Autodesk Fusion 360 part; units mm, degrees
(part 8 of 9)
equation "d1459 = ( BaseX ) + ( Wall + DeckClearance + RimBorder )"
equation "d1460 = ( BaseY + Depth + ModuleGap ) + ( ( LeftReach ) - ( ( ( ( ( LeftReach ) - ( 14 * SlotPitch + SlotWidth ) ) / 2 ) + ( 5 * SlotPitch ) ) + ( SlotWidth ) ) )"
equation "d1461 = ( LeftSideDepth ) - 2 * ( Wall + DeckClearance + RimBorder )"
equation "d1462 = SlotWidth"
equation "d1463 = DeckThick"
equation "d1465 = ( FootHeight ) + PanHeight - DeckThick"
equation "d1467 = ( BaseX ) + ( Wall + DeckClearance + RimBorder )"
equation "d1468 = ( BaseY + Depth + ModuleGap ) + ( ( LeftReach ) - ( ( ( ( ( LeftReach ) - ( 14 * SlotPitch + SlotWidth ) ) / 2 ) + ( 6 * SlotPitch ) ) + ( SlotWidth ) ) )"
equation "d1469 = ( LeftSideDepth ) - 2 * ( Wall + DeckClearance + RimBorder )"
equation "d1470 = SlotWidth"
equation "d1471 = DeckThick"
equation "d1473 = ( FootHeight ) + PanHeight - DeckThick"
equation "d1475 = ( BaseX ) + ( Wall + DeckClearance + RimBorder )"
equation "d1476 = ( BaseY + Depth + ModuleGap ) + ( ( LeftReach ) - ( ( ( ( ( LeftReach ) - ( 14 * SlotPitch + SlotWidth ) ) / 2 ) + ( 7 * SlotPitch ) ) + ( SlotWidth ) ) )"
equation "d1477 = ( LeftSideDepth ) - 2 * ( Wall + DeckClearance + RimBorder )"
equation "d1478 = SlotWidth"
equation "d1479 = DeckThick"
equation "d1481 = ( FootHeight ) + PanHeight - DeckThick"
equation "d1483 = ( BaseX ) + ( Wall + DeckClearance + RimBorder )"
equation "d1484 = ( BaseY + Depth + ModuleGap ) + ( ( LeftReach ) - ( ( ( ( ( LeftReach ) - ( 14 * SlotPitch + SlotWidth ) ) / 2 ) + ( 8 * SlotPitch ) ) + ( SlotWidth ) ) )"
equation "d1485 = ( LeftSideDepth ) - 2 * ( Wall + DeckClearance + RimBorder )"
equation "d1486 = SlotWidth"
equation "d1487 = DeckThick"
equation "d1489 = ( FootHeight ) + PanHeight - DeckThick"
equation "d1491 = ( BaseX ) + ( Wall + DeckClearance + RimBorder )"
equation "d1492 = ( BaseY + Depth + ModuleGap ) + ( ( LeftReach ) - ( ( ( ( ( LeftReach ) - ( 14 * SlotPitch + SlotWidth ) ) / 2 ) + ( 9 * SlotPitch ) ) + ( SlotWidth ) ) )"
equation "d1493 = ( LeftSideDepth ) - 2 * ( Wall + DeckClearance + RimBorder )"
equation "d1494 = SlotWidth"
equation "d1495 = DeckThick"
equation "d1497 = ( FootHeight ) + PanHeight - DeckThick"
equation "d1499 = ( BaseX ) + ( Wall + DeckClearance + RimBorder )"
equation "d1500 = ( BaseY + Depth + ModuleGap ) + ( ( LeftReach ) - ( ( ( ( ( LeftReach ) - ( 14 * SlotPitch + SlotWidth ) ) / 2 ) + ( 10 * SlotPitch ) ) + ( SlotWidth ) ) )"
equation "d1501 = ( LeftSideDepth ) - 2 * ( Wall + DeckClearance + RimBorder )"
equation "d1502 = SlotWidth"
equation "d1503 = DeckThick"
equation "d1505 = ( FootHeight ) + PanHeight - DeckThick"
equation "d1507 = ( BaseX ) + ( Wall + DeckClearance + RimBorder )"
equation "d1508 = ( BaseY + Depth + ModuleGap ) + ( ( LeftReach ) - ( ( ( ( ( LeftReach ) - ( 14 * SlotPitch + SlotWidth ) ) / 2 ) + ( 11 * SlotPitch ) ) + ( SlotWidth ) ) )"
equation "d1509 = ( LeftSideDepth ) - 2 * ( Wall + DeckClearance + RimBorder )"
equation "d1510 = SlotWidth"
equation "d1511 = DeckThick"
equation "d1513 = ( FootHeight ) + PanHeight - DeckThick"
equation "d1515 = ( BaseX ) + ( Wall + DeckClearance + RimBorder )"
equation "d1516 = ( BaseY + Depth + ModuleGap ) + ( ( LeftReach ) - ( ( ( ( ( LeftReach ) - ( 14 * SlotPitch + SlotWidth ) ) / 2 ) + ( 12 * SlotPitch ) ) + ( SlotWidth ) ) )"
equation "d1517 = ( LeftSideDepth ) - 2 * ( Wall + DeckClearance + RimBorder )"
equation "d1518 = SlotWidth"
equation "d1519 = DeckThick"
equation "d1521 = ( FootHeight ) + PanHeight - DeckThick"
equation "d1523 = ( BaseX ) + ( Wall + DeckClearance + RimBorder )"
equation "d1524 = ( BaseY + Depth + ModuleGap ) + ( ( LeftReach ) - ( ( ( ( ( LeftReach ) - ( 14 * SlotPitch + SlotWidth ) ) / 2 ) + ( 13 * SlotPitch ) ) + ( SlotWidth ) ) )"
equation "d1525 = ( LeftSideDepth ) - 2 * ( Wall + DeckClearance + RimBorder )"
equation "d1526 = SlotWidth"
equation "d1527 = DeckThick"
equation "d1529 = ( FootHeight ) + PanHeight - DeckThick"
equation "d1531 = ( BaseX ) + ( Wall + DeckClearance + RimBorder )"
equation "d1532 = ( BaseY + Depth + ModuleGap ) + ( ( LeftReach ) - ( ( ( ( ( LeftReach ) - ( 14 * SlotPitch + SlotWidth ) ) / 2 ) + ( 14 * SlotPitch ) ) + ( SlotWidth ) ) )"
equation "d1533 = ( LeftSideDepth ) - 2 * ( Wall + DeckClearance + RimBorder )"
equation "d1534 = SlotWidth"
equation "d1535 = DeckThick"
equation "d1537 = ( FootHeight ) + PanHeight - DeckThick"
equation "d1539 = ( BaseX ) + ( ( LeftSideDepth ) - Wall - DeckClearance - 4 mm )"
equation "d1540 = ( BaseY + Depth + ModuleGap ) + ( ( LeftReach ) - ( ( ( LeftReach ) / 2 - 8 mm ) + ( 16 mm ) ) )"
equation "d1543 = DeckThick"
equation "d1547 = ( BaseX ) + ( ( 11 mm ) - FootSize / 2 )"
equation "d1548 = ( BaseY + Depth + ModuleGap ) + ( ( LeftReach ) - ( ( ( 11 mm ) - FootSize / 2 ) + ( FootSize ) ) )"
equation "d1549 = FootSize"
equation "d1550 = FootSize"
equation "d1551 = FootHeight"
equation "d1553 = FootHeight"
equation "d1555 = ( BaseX ) + ( ( 11 mm ) - PegSize / 2 )"
equation "d1556 = ( BaseY + Depth + ModuleGap ) + ( ( LeftReach ) - ( ( ( 11 mm ) - PegSize / 2 ) + ( PegSize ) ) )"
equation "d1557 = PegSize"
equation "d1558 = PegSize"
equation "d1559 = PegHeight"
equation "d1563 = ( BaseX ) + ( ( ( LeftSideDepth ) - FrontFootInset ) - FootSize / 2 )"
equation "d1564 = ( BaseY + Depth + ModuleGap ) + ( ( LeftReach ) - ( ( ( 11 mm ) - FootSize / 2 ) + ( FootSize ) ) )"
equation "d1565 = FootSize"
equation "d1566 = FootSize"
equation "d1567 = FootHeight"
equation "d1569 = FootHeight"
equation "d1571 = ( BaseX ) + ( ( ( LeftSideDepth ) - FrontFootInset ) - PegSize / 2 )"
equation "d1572 = ( BaseY + Depth + ModuleGap ) + ( ( LeftReach ) - ( ( ( 11 mm ) - PegSize / 2 ) + ( PegSize ) ) )"
equation "d1573 = PegSize"
equation "d1574 = PegSize"
equation "d1575 = PegHeight"
equation "d1579 = ( BaseX ) + ( ( 11 mm ) - FootSize / 2 )"
equation "d1580 = ( BaseY + Depth + ModuleGap ) + ( ( LeftReach ) - ( ( ( ( LeftReach ) - 11 mm ) - FootSize / 2 ) + ( FootSize ) ) )"
equation "d1581 = FootSize"
equation "d1582 = FootSize"
equation "d1583 = FootHeight"
equation "d1585 = FootHeight"
equation "d1587 = ( BaseX ) + ( ( 11 mm ) - PegSize / 2 )"
equation "d1588 = ( BaseY + Depth + ModuleGap ) + ( ( LeftReach ) - ( ( ( ( LeftReach ) - 11 mm ) - PegSize / 2 ) + ( PegSize ) ) )"
equation "d1589 = PegSize"
equation "d1590 = PegSize"
equation "d1591 = PegHeight"
equation "d1595 = ( BaseX ) + ( ( ( LeftSideDepth ) - FrontFootInset ) - FootSize / 2 )"
equation "d1596 = ( BaseY + Depth + ModuleGap ) + ( ( LeftReach ) - ( ( ( ( LeftReach ) - 11 mm ) - FootSize / 2 ) + ( FootSize ) ) )"
equation "d1597 = FootSize"
equation "d1598 = FootSize"
equation "d1599 = FootHeight"
equation "d1601 = FootHeight"
equation "d1603 = ( BaseX ) + ( ( ( LeftSideDepth ) - FrontFootInset ) - PegSize / 2 )"
equation "d1604 = ( BaseY + Depth + ModuleGap ) + ( ( LeftReach ) - ( ( ( ( LeftReach ) - 11 mm ) - PegSize / 2 ) + ( PegSize ) ) )"
equation "d1605 = PegSize"
equation "d1606 = PegSize"
equation "d1607 = PegHeight"
equation "d1609 = FootHeight"
equation "d1611 = ( BaseX + LeftRun + FaucetGap + RightRun - RightSideDepth ) + ( ( RightSideDepth ) - ( ( 0 mm ) + ( RightSideDepth ) ) )"
equation "d1612 = ( BaseY + Depth + ModuleGap ) + ( 0 mm )"
equation "d1613 = RightSideDepth"
equation "d1614 = RightReach"
equation "d1615 = PanHeight"
equation "d1619 = ( BaseY + Depth + ModuleGap ) + ( Wall )"
equation "d1621 = ( ( BaseX + LeftRun + FaucetGap + RightRun - RightSideDepth ) + ( ( RightSideDepth ) - ( Wall ) ) )"
equation "d1622 = -( -( ( FootHeight ) + FloorMin + DrainExtension * tan(DrainSlope) + ( ( RightSideDepth ) - ( Wall ) ) * tan(DrainSlope) ) )"
equation "d1623 = ( ( BaseX + LeftRun + FaucetGap + RightRun - RightSideDepth ) + ( ( RightSideDepth ) - ( ( RightSideDepth ) - Wall ) ) )"
equation "d1624 = -( -( ( FootHeight ) + FloorMin + DrainExtension * tan(DrainSlope) + ( ( RightSideDepth ) - ( ( RightSideDepth ) - Wall ) ) * tan(DrainSlope) ) )"
equation "d1625 = -( -( ( FootHeight ) + PanHeight + 1 mm ) )"
equation "d1626 = ( RightReach ) - 2 * Wall"
equation "d1628 = ( BaseY + Depth + ModuleGap ) + ( ( RightReach / 2 ) - DrainWidth / 2 - Wall )"
equation "d1630 = ( ( BaseX + LeftRun + FaucetGap + RightRun - RightSideDepth ) + ( ( RightSideDepth ) - ( ( RightSideDepth ) - Wall ) ) )"
equation "d1631 = -( -( FootHeight ) )"
equation "d1632 = ( ( BaseX + LeftRun + FaucetGap + RightRun - RightSideDepth ) + ( ( RightSideDepth ) - ( ( RightSideDepth ) + DrainExtension ) ) )"
equation "d1633 = -( -( ( FootHeight ) + FloorMin + DrainExtension * tan(DrainSlope) + ( ( RightSideDepth ) - ( ( RightSideDepth ) + DrainExtension ) ) * tan(DrainSlope) ) )"
equation "d1634 = -( -( ( FootHeight ) + FloorMin + DrainExtension * tan(DrainSlope) + ( ( RightSideDepth ) - ( ( RightSideDepth ) - Wall ) ) * tan(DrainSlope) ) )"
equation "d1635 = DrainWidth + 2 * Wall"
equation "d1637 = ( BaseY + Depth + ModuleGap ) + ( ( RightReach / 2 ) - DrainWidth / 2 - Wall )"
equation "d1639 = ( ( BaseX + LeftRun + FaucetGap + RightRun - RightSideDepth ) + ( ( RightSideDepth ) - ( ( RightSideDepth ) - Wall ) ) )"
equation "d1640 = -( -( FootHeight ) )"
equation "d1641 = ( ( BaseX + LeftRun + FaucetGap + RightRun - RightSideDepth ) + ( ( RightSideDepth ) - ( ( RightSideDepth ) + DrainExtension ) ) )"
equation "d1642 = -( -( ( ( FootHeight ) + FloorMin + DrainExtension * tan(DrainSlope) + ( ( RightSideDepth ) - ( ( RightSideDepth ) + DrainExtension ) ) * tan(DrainSlope) ) + ( 6 mm ) ) )"
equation "d1643 = -( -( ( ( FootHeight ) + FloorMin + DrainExtension * tan(DrainSlope) + ( ( RightSideDepth ) - ( ( RightSideDepth ) - Wall ) ) * tan(DrainSlope) ) + ( 6 mm ) ) )"
equation "d1644 = Wall"
equation "d1646 = ( BaseY + Depth + ModuleGap ) + ( ( RightReach / 2 ) + DrainWidth / 2 )"
equation "d1648 = ( ( BaseX + LeftRun + FaucetGap + RightRun - RightSideDepth ) + ( ( RightSideDepth ) - ( ( RightSideDepth ) - Wall ) ) )"
equation "d1649 = -( -( FootHeight ) )"
equation "d1650 = ( ( BaseX + LeftRun + FaucetGap + RightRun - RightSideDepth ) + ( ( RightSideDepth ) - ( ( RightSideDepth ) + DrainExtension ) ) )"
equation "d1651 = -( -( ( ( FootHeight ) + FloorMin + DrainExtension * tan(DrainSlope) + ( ( RightSideDepth ) - ( ( RightSideDepth ) + DrainExtension ) ) * tan(DrainSlope) ) + ( 6 mm ) ) )"
equation "d1652 = -( -( ( ( FootHeight ) + FloorMin + DrainExtension * tan(DrainSlope) + ( ( RightSideDepth ) - ( ( RightSideDepth ) - Wall ) ) * tan(DrainSlope) ) + ( 6 mm ) ) )"
equation "d1653 = Wall"
equation "d1655 = ( BaseY + Depth + ModuleGap ) + ( ( RightReach / 2 ) - DrainWidth / 2 )"
equation "d1657 = ( ( BaseX + LeftRun + FaucetGap + RightRun - RightSideDepth ) + ( ( RightSideDepth ) - ( ( RightSideDepth ) - Wall ) ) )"
equation "d1658 = -( -( ( FootHeight ) + FloorMin + DrainExtension * tan(DrainSlope) + ( ( RightSideDepth ) - ( ( RightSideDepth ) - Wall ) ) * tan(DrainSlope) ) )"
equation "d1659 = ( ( BaseX + LeftRun + FaucetGap + RightRun - RightSideDepth ) + ( ( RightSideDepth ) - ( ( RightSideDepth ) + DrainExtension ) ) )"
equation "d1660 = -( -( ( FootHeight ) + FloorMin + DrainExtension * tan(DrainSlope) + ( ( RightSideDepth ) - ( ( RightSideDepth ) + DrainExtension ) ) * tan(DrainSlope) ) )"
equation "d1661 = -( -( ( FootHeight ) + PanHeight + 1 mm ) )"
equation "d1662 = DrainWidth"
equation "d1664 = FootHeight"
equation "d1666 = ( BaseX + LeftRun + FaucetGap + RightRun - RightSideDepth ) + ( ( RightSideDepth ) - ( ( Wall ) + ( 12 mm ) ) )"
equation "d1667 = ( BaseY + Depth + ModuleGap ) + ( Wall )"
equation "d1670 = PanHeight - DeckThick"
equation "d1672 = FootHeight"
equation "d1674 = ( BaseX + LeftRun + FaucetGap + RightRun - RightSideDepth ) + ( ( RightSideDepth ) - ( ( ( RightSideDepth ) - Wall - 12 mm ) + ( 12 mm ) ) )"
equation "d1675 = ( BaseY + Depth + ModuleGap ) + ( Wall )"
equation "d1678 = PanHeight - DeckThick"
equation "d1680 = FootHeight"
equation "d1682 = ( BaseX + LeftRun + FaucetGap + RightRun - RightSideDepth ) + ( ( RightSideDepth ) - ( ( Wall ) + ( 12 mm ) ) )"
equation "d1683 = ( BaseY + Depth + ModuleGap ) + ( ( RightReach ) - Wall - 12 mm )"
equation "d1686 = PanHeight - DeckThick"
equation "d1688 = FootHeight"
equation "d1690 = ( BaseX + LeftRun + FaucetGap + RightRun - RightSideDepth ) + ( ( RightSideDepth ) - ( ( ( RightSideDepth ) - Wall - 12 mm ) + ( 12 mm ) ) )"
equation "d1691 = ( BaseY + Depth + ModuleGap ) + ( ( RightReach ) - Wall - 12 mm )"
equation "d1694 = PanHeight - DeckThick"
equation "d1696 = ( BaseY + Depth + ModuleGap ) + ( ( RightReach / 2 ) - DrainWidth / 2 - Wall )"
equation "d1698 = ( ( BaseX + LeftRun + FaucetGap + RightRun - RightSideDepth ) + ( ( RightSideDepth ) - ( ( RightSideDepth ) + DrainExtension - 2 mm ) ) )"
equation "d1699 = -( -( ( FootHeight ) - ( 0.2 mm ) ) )"
equation "d1700 = ( ( BaseX + LeftRun + FaucetGap + RightRun - RightSideDepth ) + ( ( RightSideDepth ) - ( ( ( RightSideDepth ) + DrainExtension - 2 mm ) + ( 1 mm ) ) ) )"
equation "d1701 = -( -( ( FootHeight ) + ( 0.6 mm ) ) )"
equation "d1702 = DrainWidth + 2 * Wall"
equation "d1704 = FootHeight"
equation "d1706 = ( BaseX + LeftRun + FaucetGap + RightRun - RightSideDepth ) + ( ( RightSideDepth ) - ( ( ( 11 mm ) - PegSize / 2 - FitClearance ) + ( PegSize + 2 * FitClearance ) ) )"
equation "d1707 = ( BaseY + Depth + ModuleGap ) + ( ( 11 mm ) - PegSize / 2 - FitClearance )"
equation "d1708 = PegSize + 2 * FitClearance"
equation "d1709 = PegSize + 2 * FitClearance"
equation "d1710 = PegHeight + 0.3 mm"
equation "d1712 = FootHeight"
equation "d1714 = ( BaseX + LeftRun + FaucetGap + RightRun - RightSideDepth ) + ( ( RightSideDepth ) - ( ( ( ( RightSideDepth ) - FrontFootInset ) - PegSize / 2 - FitClearance ) + ( PegSize + 2 * FitClearance ) ) )"
equation "d1715 = ( BaseY + Depth + ModuleGap ) + ( ( 11 mm ) - PegSize / 2 - FitClearance )"
equation "d1716 = PegSize + 2 * FitClearance"
equation "d1717 = PegSize + 2 * FitClearance"
equation "d1718 = PegHeight + 0.3 mm"
equation "d1720 = FootHeight"
equation "d1722 = ( BaseX + LeftRun + FaucetGap + RightRun - RightSideDepth ) + ( ( RightSideDepth ) - ( ( ( 11 mm ) - PegSize / 2 - FitClearance ) + ( PegSize + 2 * FitClearance ) ) )"
equation "d1723 = ( BaseY + Depth + ModuleGap ) + ( ( ( RightReach ) - 11 mm ) - PegSize / 2 - FitClearance )"
equation "d1724 = PegSize + 2 * FitClearance"
equation "d1725 = PegSize + 2 * FitClearance"
equation "d1726 = PegHeight + 0.3 mm"
equation "d1728 = FootHeight"
equation "d1730 = ( BaseX + LeftRun + FaucetGap + RightRun - RightSideDepth ) + ( ( RightSideDepth ) - ( ( ( ( RightSideDepth ) - FrontFootInset ) - PegSize / 2 - FitClearance ) + ( PegSize + 2 * FitClearance ) ) )"
equation "d1731 = ( BaseY + Depth + ModuleGap ) + ( ( ( RightReach ) - 11 mm ) - PegSize / 2 - FitClearance )"
equation "d1732 = PegSize + 2 * FitClearance"
equation "d1733 = PegSize + 2 * FitClearance"
equation "d1734 = PegHeight + 0.3 mm"
equation "d1736 = ( FootHeight ) + PanHeight - DeckThick"
equation "d1738 = ( BaseX + LeftRun + FaucetGap + RightRun - RightSideDepth ) + ( ( RightSideDepth ) - ( ( Wall + DeckClearance ) + ( ( RightSideDepth ) - 2 * ( Wall + DeckClearance ) ) ) )"
equation "d1739 = ( BaseY + Depth + ModuleGap ) + ( Wall + DeckClearance )"
equation "d1740 = ( RightSideDepth ) - 2 * ( Wall + DeckClearance )"
equation "d1741 = ( RightReach ) - 2 * ( Wall + DeckClearance )"
equation "d1742 = DeckThick"
equation "d1744 = ( FootHeight ) + PanHeight - DeckThick"
equation "d1746 = ( BaseX + LeftRun + FaucetGap + RightRun - RightSideDepth ) + ( ( RightSideDepth ) - ( ( Wall + DeckClearance + RimBorder ) + ( ( RightSideDepth ) - 2 * ( Wall + DeckClearance + RimBorder ) ) ) )"
equation "d1747 = ( BaseY + Depth + ModuleGap ) + ( ( ( ( RightReach ) - ( 14 * SlotPitch + SlotWidth ) ) / 2 ) + ( 0 * SlotPitch ) )"
equation "d1748 = ( RightSideDepth ) - 2 * ( Wall + DeckClearance + RimBorder )"
equation "d1749 = SlotWidth"
equation "d1750 = DeckThick"
equation "d1752 = ( FootHeight ) + PanHeight - DeckThick"
equation "d1754 = ( BaseX + LeftRun + FaucetGap + RightRun - RightSideDepth ) + ( ( RightSideDepth ) - ( ( Wall + DeckClearance + RimBorder ) + ( ( RightSideDepth ) - 2 * ( Wall + DeckClearance + RimBorder ) ) ) )"
equation "d1755 = ( BaseY + Depth + ModuleGap ) + ( ( ( ( RightReach ) - ( 14 * SlotPitch + SlotWidth ) ) / 2 ) + ( 1 * SlotPitch ) )"
equation "d1756 = ( RightSideDepth ) - 2 * ( Wall + DeckClearance + RimBorder )"
equation "d1757 = SlotWidth"
equation "d1758 = DeckThick"
equation "d1760 = ( FootHeight ) + PanHeight - DeckThick"
equation "d1762 = ( BaseX + LeftRun + FaucetGap + RightRun - RightSideDepth ) + ( ( RightSideDepth ) - ( ( Wall + DeckClearance + RimBorder ) + ( ( RightSideDepth ) - 2 * ( Wall + DeckClearance + RimBorder ) ) ) )"
equation "d1763 = ( BaseY + Depth + ModuleGap ) + ( ( ( ( RightReach ) - ( 14 * SlotPitch + SlotWidth ) ) / 2 ) + ( 2 * SlotPitch ) )"
equation "d1764 = ( RightSideDepth ) - 2 * ( Wall + DeckClearance + RimBorder )"
equation "d1765 = SlotWidth"
equation "d1766 = DeckThick"
equation "d1768 = ( FootHeight ) + PanHeight - DeckThick"
equation "d1770 = ( BaseX + LeftRun + FaucetGap + RightRun - RightSideDepth ) + ( ( RightSideDepth ) - ( ( Wall + DeckClearance + RimBorder ) + ( ( RightSideDepth ) - 2 * ( Wall + DeckClearance + RimBorder ) ) ) )"
equation "d1771 = ( BaseY + Depth + ModuleGap ) + ( ( ( ( RightReach ) - ( 14 * SlotPitch + SlotWidth ) ) / 2 ) + ( 3 * SlotPitch ) )"
equation "d1772 = ( RightSideDepth ) - 2 * ( Wall + DeckClearance + RimBorder )"
equation "d1773 = SlotWidth"
equation "d1774 = DeckThick"
equation "d1776 = ( FootHeight ) + PanHeight - DeckThick"
equation "d1778 = ( BaseX + LeftRun + FaucetGap + RightRun - RightSideDepth ) + ( ( RightSideDepth ) - ( ( Wall + DeckClearance + RimBorder ) + ( ( RightSideDepth ) - 2 * ( Wall + DeckClearance + RimBorder ) ) ) )"
equation "d1779 = ( BaseY + Depth + ModuleGap ) + ( ( ( ( RightReach ) - ( 14 * SlotPitch + SlotWidth ) ) / 2 ) + ( 4 * SlotPitch ) )"
equation "d1780 = ( RightSideDepth ) - 2 * ( Wall + DeckClearance + RimBorder )"
equation "d1781 = SlotWidth"
equation "d1782 = DeckThick"
equation "d1784 = ( FootHeight ) + PanHeight - DeckThick"
equation "d1786 = ( BaseX + LeftRun + FaucetGap + RightRun - RightSideDepth ) + ( ( RightSideDepth ) - ( ( Wall + DeckClearance + RimBorder ) + ( ( RightSideDepth ) - 2 * ( Wall + DeckClearance + RimBorder ) ) ) )"
equation "d1787 = ( BaseY + Depth + ModuleGap ) + ( ( ( ( RightReach ) - ( 14 * SlotPitch + SlotWidth ) ) / 2 ) + ( 5 * SlotPitch ) )"
equation "d1788 = ( RightSideDepth ) - 2 * ( Wall + DeckClearance + RimBorder )"
equation "d1789 = SlotWidth"
equation "d1790 = DeckThick"
equation "d1792 = ( FootHeight ) + PanHeight - DeckThick"
equation "d1794 = ( BaseX + LeftRun + FaucetGap + RightRun - RightSideDepth ) + ( ( RightSideDepth ) - ( ( Wall + DeckClearance + RimBorder ) + ( ( RightSideDepth ) - 2 * ( Wall + DeckClearance + RimBorder ) ) ) )"
equation "d1795 = ( BaseY + Depth + ModuleGap ) + ( ( ( ( RightReach ) - ( 14 * SlotPitch + SlotWidth ) ) / 2 ) + ( 6 * SlotPitch ) )"
equation "d1796 = ( RightSideDepth ) - 2 * ( Wall + DeckClearance + RimBorder )"
equation "d1797 = SlotWidth"
equation "d1798 = DeckThick"
equation "d1800 = ( FootHeight ) + PanHeight - DeckThick"
equation "d1802 = ( BaseX + LeftRun + FaucetGap + RightRun - RightSideDepth ) + ( ( RightSideDepth ) - ( ( Wall + DeckClearance + RimBorder ) + ( ( RightSideDepth ) - 2 * ( Wall + DeckClearance + RimBorder ) ) ) )"
equation "d1803 = ( BaseY + Depth + ModuleGap ) + ( ( ( ( RightReach ) - ( 14 * SlotPitch + SlotWidth ) ) / 2 ) + ( 7 * SlotPitch ) )"
equation "d1804 = ( RightSideDepth ) - 2 * ( Wall + DeckClearance + RimBorder )"
equation "d1805 = SlotWidth"
equation "d1806 = DeckThick"
equation "d1808 = ( FootHeight ) + PanHeight - DeckThick"
equation "d1810 = ( BaseX + LeftRun + FaucetGap + RightRun - RightSideDepth ) + ( ( RightSideDepth ) - ( ( Wall + DeckClearance + RimBorder ) + ( ( RightSideDepth ) - 2 * ( Wall + DeckClearance + RimBorder ) ) ) )"
equation "d1811 = ( BaseY + Depth + ModuleGap ) + ( ( ( ( RightReach ) - ( 14 * SlotPitch + SlotWidth ) ) / 2 ) + ( 8 * SlotPitch ) )"
equation "d1812 = ( RightSideDepth ) - 2 * ( Wall + DeckClearance + RimBorder )"
equation "d1813 = SlotWidth"
equation "d1814 = DeckThick"
equation "d1816 = ( FootHeight ) + PanHeight - DeckThick"
equation "d1818 = ( BaseX + LeftRun + FaucetGap + RightRun - RightSideDepth ) + ( ( RightSideDepth ) - ( ( Wall + DeckClearance + RimBorder ) + ( ( RightSideDepth ) - 2 * ( Wall + DeckClearance + RimBorder ) ) ) )"
equation "d1819 = ( BaseY + Depth + ModuleGap ) + ( ( ( ( RightReach ) - ( 14 * SlotPitch + SlotWidth ) ) / 2 ) + ( 9 * SlotPitch ) )"
equation "d1820 = ( RightSideDepth ) - 2 * ( Wall + DeckClearance + RimBorder )"
equation "d1821 = SlotWidth"
equation "d1822 = DeckThick"
equation "d1824 = ( FootHeight ) + PanHeight - DeckThick"
equation "d1826 = ( BaseX + LeftRun + FaucetGap + RightRun - RightSideDepth ) + ( ( RightSideDepth ) - ( ( Wall + DeckClearance + RimBorder ) + ( ( RightSideDepth ) - 2 * ( Wall + DeckClearance + RimBorder ) ) ) )"
equation "d1827 = ( BaseY + Depth + ModuleGap ) + ( ( ( ( RightReach ) - ( 14 * SlotPitch + SlotWidth ) ) / 2 ) + ( 10 * SlotPitch ) )"
equation "d1828 = ( RightSideDepth ) - 2 * ( Wall + DeckClearance + RimBorder )"
equation "d1829 = SlotWidth"
equation "d1830 = DeckThick"
equation "d1832 = ( FootHeight ) + PanHeight - DeckThick"
equation "d1834 = ( BaseX + LeftRun + FaucetGap + RightRun - RightSideDepth ) + ( ( RightSideDepth ) - ( ( Wall + DeckClearance + RimBorder ) + ( ( RightSideDepth ) - 2 * ( Wall + DeckClearance + RimBorder ) ) ) )"
equation "d1835 = ( BaseY + Depth + ModuleGap ) + ( ( ( ( RightReach ) - ( 14 * SlotPitch + SlotWidth ) ) / 2 ) + ( 11 * SlotPitch ) )"
equation "d1836 = ( RightSideDepth ) - 2 * ( Wall + DeckClearance + RimBorder )"
equation "d1837 = SlotWidth"
equation "d1838 = DeckThick"
equation "d1840 = ( FootHeight ) + PanHeight - DeckThick"
equation "d1842 = ( BaseX + LeftRun + FaucetGap + RightRun - RightSideDepth ) + ( ( RightSideDepth ) - ( ( Wall + DeckClearance + RimBorder ) + ( ( RightSideDepth ) - 2 * ( Wall + DeckClearance + RimBorder ) ) ) )"
equation "d1843 = ( BaseY + Depth + ModuleGap ) + ( ( ( ( RightReach ) - ( 14 * SlotPitch + SlotWidth ) ) / 2 ) + ( 12 * SlotPitch ) )"
equation "d1844 = ( RightSideDepth ) - 2 * ( Wall + DeckClearance + RimBorder )"
equation "d1845 = SlotWidth"
equation "d1846 = DeckThick"
equation "d1848 = ( FootHeight ) + PanHeight - DeckThick"
equation "d1850 = ( BaseX + LeftRun + FaucetGap + RightRun - RightSideDepth ) + ( ( RightSideDepth ) - ( ( Wall + DeckClearance + RimBorder ) + ( ( RightSideDepth ) - 2 * ( Wall + DeckClearance + RimBorder ) ) ) )"
equation "d1851 = ( BaseY + Depth + ModuleGap ) + ( ( ( ( RightReach ) - ( 14 * SlotPitch + SlotWidth ) ) / 2 ) + ( 13 * SlotPitch ) )"
equation "d1852 = ( RightSideDepth ) - 2 * ( Wall + DeckClearance + RimBorder )"
equation "d1853 = SlotWidth"
equation "d1854 = DeckThick"
equation "d1856 = ( FootHeight ) + PanHeight - DeckThick"
equation "d1858 = ( BaseX + LeftRun + FaucetGap + RightRun - RightSideDepth ) + ( ( RightSideDepth ) - ( ( Wall + DeckClearance + RimBorder ) + ( ( RightSideDepth ) - 2 * ( Wall + DeckClearance + RimBorder ) ) ) )"
equation "d1859 = ( BaseY + Depth + ModuleGap ) + ( ( ( ( RightReach ) - ( 14 * SlotPitch + SlotWidth ) ) / 2 ) + ( 14 * SlotPitch ) )"
equation "d1860 = ( RightSideDepth ) - 2 * ( Wall + DeckClearance + RimBorder )"
equation "d1861 = SlotWidth"
equation "d1862 = DeckThick"
equation "d1864 = ( FootHeight ) + PanHeight - DeckThick"
equation "d1866 = ( BaseX + LeftRun + FaucetGap + RightRun - RightSideDepth ) + ( ( RightSideDepth ) - ( ( ( RightSideDepth ) - Wall - DeckClearance - 4 mm ) + ( 5 mm ) ) )"
equation "d1867 = ( BaseY + Depth + ModuleGap ) + ( ( RightReach ) / 2 - 8 mm )"
equation "d1870 = DeckThick"
equation "d1874 = ( BaseX + LeftRun + FaucetGap + RightRun - RightSideDepth ) + ( ( RightSideDepth ) - ( ( ( 11 mm ) - FootSize / 2 ) + ( FootSize ) ) )"
equation "d1875 = ( BaseY + Depth + ModuleGap ) + ( ( 11 mm ) - FootSize / 2 )"
equation "d1876 = FootSize"
equation "d1877 = FootSize"
equation "d1878 = FootHeight"
equation "d1880 = FootHeight"
equation "d1882 = ( BaseX + LeftRun + FaucetGap + RightRun - RightSideDepth ) + ( ( RightSideDepth ) - ( ( ( 11 mm ) - PegSize / 2 ) + ( PegSize ) ) )"
equation "d1883 = ( BaseY + Depth + ModuleGap ) + ( ( 11 mm ) - PegSize / 2 )"
equation "d1884 = PegSize"
equation "d1885 = PegSize"
equation "d1886 = PegHeight"
equation "d1890 = ( BaseX + LeftRun + FaucetGap + RightRun - RightSideDepth ) + ( ( RightSideDepth ) - ( ( ( ( RightSideDepth ) - FrontFootInset ) - FootSize / 2 ) + ( FootSize ) ) )"
equation "d1891 = ( BaseY + Depth + ModuleGap ) + ( ( 11 mm ) - FootSize / 2 )"
equation "d1892 = FootSize"
equation "d1893 = FootSize"
equation "d1894 = FootHeight"
equation "d1896 = FootHeight"
equation "d1898 = ( BaseX + LeftRun + FaucetGap + RightRun - RightSideDepth ) + ( ( RightSideDepth ) - ( ( ( ( RightSideDepth ) - FrontFootInset ) - PegSize / 2 ) + ( PegSize ) ) )"
equation "d1899 = ( BaseY + Depth + ModuleGap ) + ( ( 11 mm ) - PegSize / 2 )"
equation "d1900 = PegSize"
equation "d1901 = PegSize"
equation "d1902 = PegHeight"
equation "d1906 = ( BaseX + LeftRun + FaucetGap + RightRun - RightSideDepth ) + ( ( RightSideDepth ) - ( ( ( 11 mm ) - FootSize / 2 ) + ( FootSize ) ) )"
equation "d1907 = ( BaseY + Depth + ModuleGap ) + ( ( ( RightReach ) - 11 mm ) - FootSize / 2 )"
equation "d1908 = FootSize"
equation "d1909 = FootSize"
equation "d1910 = FootHeight"
equation "d1912 = FootHeight"
equation "d1914 = ( BaseX + LeftRun + FaucetGap + RightRun - RightSideDepth ) + ( ( RightSideDepth ) - ( ( ( 11 mm ) - PegSize / 2 ) + ( PegSize ) ) )"
equation "d1915 = ( BaseY + Depth + ModuleGap ) + ( ( ( RightReach ) - 11 mm ) - PegSize / 2 )"
equation "d1916 = PegSize"
equation "d1917 = PegSize"
equation "d1918 = PegHeight"
equation "d1922 = ( BaseX + LeftRun + FaucetGap + RightRun - RightSideDepth ) + ( ( RightSideDepth ) - ( ( ( ( RightSideDepth ) - FrontFootInset ) - FootSize / 2 ) + ( FootSize ) ) )"
equation "d1923 = ( BaseY + Depth + ModuleGap ) + ( ( ( RightReach ) - 11 mm ) - FootSize / 2 )"
equation "d1924 = FootSize"
equation "d1925 = FootSize"
equation "d1926 = FootHeight"
equation "d1928 = FootHeight"
equation "d1930 = ( BaseX + LeftRun + FaucetGap + RightRun - RightSideDepth ) + ( ( RightSideDepth ) - ( ( ( ( RightSideDepth ) - FrontFootInset ) - PegSize / 2 ) + ( PegSize ) ) )"
equation "d1931 = ( BaseY + Depth + ModuleGap ) + ( ( ( RightReach ) - 11 mm ) - PegSize / 2 )"
equation "d1932 = PegSize"
equation "d1933 = PegSize"
equation "d1934 = PegHeight"
equation "d1936 = UpperDeckHeight - PanHeight"
equation "d1938 = ( BaseX ) + ( 0 mm )"
equation "d1939 = ( BaseY ) + ( 0 mm )"
equation "d1940 = TowerWidth"
equation "d1941 = Depth"
equation "d1942 = PanHeight"
equation "d1946 = ( BaseX ) + ( Wall )"
equation "d1948 = -( -( ( UpperDeckHeight - PanHeight ) + FloorMin + DrainExtension * tan(DrainSlope) + ( ( Depth ) - ( Wall ) ) * tan(DrainSlope) ) )"
equation "d1949 = ( ( BaseY ) + ( Wall ) )"
equation "d1950 = -( -( ( UpperDeckHeight - PanHeight ) + FloorMin + DrainExtension * tan(DrainSlope) + ( ( Depth ) - ( ( Depth ) - Wall ) ) * tan(DrainSlope) ) )"
equation "d1951 = ( ( BaseY ) + ( ( Depth ) - Wall ) )"
equation "d1952 = -( -( ( UpperDeckHeight - PanHeight ) + PanHeight + 1 mm ) )"
equation "d1953 = ( TowerWidth ) - 2 * Wall"
equation "d1955 = ( BaseX ) + ( ( TowerWidth - 35 mm ) - DrainWidth / 2 - Wall )"
equation "d1957 = -( -( UpperDeckHeight - PanHeight ) )"
equation "d1958 = ( ( BaseY ) + ( ( Depth ) - Wall ) )"
equation "d1959 = ( ( BaseY ) + ( ( Depth ) + DrainExtension ) )"
equation "d1960 = -( -( ( UpperDeckHeight - PanHeight ) + FloorMin + DrainExtension * tan(DrainSlope) + ( ( Depth ) - ( ( Depth ) + DrainExtension ) ) * tan(DrainSlope) ) )"
equation "d1961 = -( -( ( UpperDeckHeight - PanHeight ) + FloorMin + DrainExtension * tan(DrainSlope) + ( ( Depth ) - ( ( Depth ) - Wall ) ) * tan(DrainSlope) ) )"
equation "d1962 = DrainWidth + 2 * Wall"
equation "d1964 = ( BaseX ) + ( ( TowerWidth - 35 mm ) - DrainWidth / 2 - Wall )"
equation "d1966 = -( -( UpperDeckHeight - PanHeight ) )"
equation "d1967 = ( ( BaseY ) + ( ( Depth ) - Wall ) )"
equation "d1968 = ( ( BaseY ) + ( ( Depth ) + DrainExtension ) )"
equation "d1969 = -( -( ( ( UpperDeckHeight - PanHeight ) + FloorMin + DrainExtension * tan(DrainSlope) + ( ( Depth ) - ( ( Depth ) + DrainExtension ) ) * tan(DrainSlope) ) + ( 6 mm ) ) )"
equation "d1970 = -( -( ( ( UpperDeckHeight - PanHeight ) + FloorMin + DrainExtension * tan(DrainSlope) + ( ( Depth ) - ( ( Depth ) - Wall ) ) * tan(DrainSlope) ) + ( 6 mm ) ) )"
equation "d1971 = Wall"
equation "d1973 = ( BaseX ) + ( ( TowerWidth - 35 mm ) + DrainWidth / 2 )"
equation "d1975 = -( -( UpperDeckHeight - PanHeight ) )"
equation "d1976 = ( ( BaseY ) + ( ( Depth ) - Wall ) )"
equation "d1977 = ( ( BaseY ) + ( ( Depth ) + DrainExtension ) )"
equation "d1978 = -( -( ( ( UpperDeckHeight - PanHeight ) + FloorMin + DrainExtension * tan(DrainSlope) + ( ( Depth ) - ( ( Depth ) + DrainExtension ) ) * tan(DrainSlope) ) + ( 6 mm ) ) )"
equation "d1979 = -( -( ( ( UpperDeckHeight - PanHeight ) + FloorMin + DrainExtension * tan(DrainSlope) + ( ( Depth ) - ( ( Depth ) - Wall ) ) * tan(DrainSlope) ) + ( 6 mm ) ) )"
equation "d1980 = Wall"
equation "d1982 = ( BaseX ) + ( ( TowerWidth - 35 mm ) - DrainWidth / 2 )"
equation "d1984 = -( -( ( UpperDeckHeight - PanHeight ) + FloorMin + DrainExtension * tan(DrainSlope) + ( ( Depth ) - ( ( Depth ) - Wall ) ) * tan(DrainSlope) ) )"
equation "d1985 = ( ( BaseY ) + ( ( Depth ) - Wall ) )"
equation "d1986 = -( -( ( UpperDeckHeight - PanHeight ) + FloorMin + DrainExtension * tan(DrainSlope) + ( ( Depth ) - ( ( Depth ) + DrainExtension ) ) * tan(DrainSlope) ) )"
equation "d1987 = ( ( BaseY ) + ( ( Depth ) + DrainExtension ) )"
equation "d1988 = -( -( ( UpperDeckHeight - PanHeight ) + PanHeight + 1 mm ) )"
equation "d1989 = DrainWidth"
equation "d1991 = UpperDeckHeight - PanHeight"
equation "d1993 = ( BaseX ) + ( Wall )"
equation "d1994 = ( BaseY ) + ( Wall )"
equation "d1997 = PanHeight - DeckThick"
equation "d1999 = UpperDeckHeight - PanHeight"
equation "d2001 = ( BaseX ) + ( Wall )"
equation "d2002 = ( BaseY ) + ( ( Depth ) - Wall - 12 mm )"
equation "d2005 = PanHeight - DeckThick"
equation "d2007 = UpperDeckHeight - PanHeight"
equation "d2009 = ( BaseX ) + ( ( TowerWidth ) - Wall - 12 mm )"
equation "d2010 = ( BaseY ) + ( Wall )"
equation "d2013 = PanHeight - DeckThick"
equation "d2015 = UpperDeckHeight - PanHeight"
equation "d2017 = ( BaseX ) + ( ( TowerWidth ) - Wall - 12 mm )"
equation "d2018 = ( BaseY ) + ( ( Depth ) - Wall - 12 mm )"
equation "d2021 = PanHeight - DeckThick"
equation "d2023 = ( BaseX ) + ( ( TowerWidth - 35 mm ) - DrainWidth / 2 - Wall )"
equation "d2025 = -( -( ( UpperDeckHeight - PanHeight ) - ( 0.2 mm ) ) )"
equation "d2026 = ( ( BaseY ) + ( ( Depth ) + DrainExtension - 2 mm ) )"
equation "d2027 = ( ( BaseY ) + ( ( ( Depth ) + DrainExtension - 2 mm ) + ( 1 mm ) ) )"
equation "d2028 = -( -( ( UpperDeckHeight - PanHeight ) + ( 0.6 mm ) ) )"
equation "d2029 = DrainWidth + 2 * Wall"
equation "d2031 = ( UpperDeckHeight - PanHeight ) + PanHeight - DeckThick"
equation "d2033 = ( BaseX ) + ( Wall + DeckClearance )"
equation "d2034 = ( BaseY ) + ( Wall + DeckClearance )"
equation "d2035 = ( TowerWidth ) - 2 * ( Wall + DeckClearance )"
equation "d2036 = ( Depth ) - 2 * ( Wall + DeckClearance )"
equation "d2037 = DeckThick"
equation "d2039 = ( UpperDeckHeight - PanHeight ) + PanHeight - DeckThick"
equation "d2041 = ( BaseX ) + ( ( ( ( TowerWidth ) - ( 14 * SlotPitch + SlotWidth ) ) / 2 ) + ( 0 * SlotPitch ) )"
equation "d2042 = ( BaseY ) + ( Wall + DeckClearance + RimBorder )"
equation "d2043 = SlotWidth"
equation "d2044 = ( Depth ) - 2 * ( Wall + DeckClearance + RimBorder )"
equation "d2045 = DeckThick"
equation "d2047 = ( UpperDeckHeight - PanHeight ) + PanHeight - DeckThick"
equation "d2049 = ( BaseX ) + ( ( ( ( TowerWidth ) - ( 14 * SlotPitch + SlotWidth ) ) / 2 ) + ( 1 * SlotPitch ) )"
equation "d2050 = ( BaseY ) + ( Wall + DeckClearance + RimBorder )"
equation "d2051 = SlotWidth"
equation "d2052 = ( Depth ) - 2 * ( Wall + DeckClearance + RimBorder )"
equation "d2053 = DeckThick"
equation "d2055 = ( UpperDeckHeight - PanHeight ) + PanHeight - DeckThick"
equation "d2057 = ( BaseX ) + ( ( ( ( TowerWidth ) - ( 14 * SlotPitch + SlotWidth ) ) / 2 ) + ( 2 * SlotPitch ) )"
equation "d2058 = ( BaseY ) + ( Wall + DeckClearance + RimBorder )"
equation "d2059 = SlotWidth"
equation "d2060 = ( Depth ) - 2 * ( Wall + DeckClearance + RimBorder )"
equation "d2061 = DeckThick"
equation "d2063 = ( UpperDeckHeight - PanHeight ) + PanHeight - DeckThick"
equation "d2065 = ( BaseX ) + ( ( ( ( TowerWidth ) - ( 14 * SlotPitch + SlotWidth ) ) / 2 ) + ( 3 * SlotPitch ) )"
equation "d2066 = ( BaseY ) + ( Wall + DeckClearance + RimBorder )"
equation "d2067 = SlotWidth"
equation "d2068 = ( Depth ) - 2 * ( Wall + DeckClearance + RimBorder )"
equation "d2069 = DeckThick"
equation "d2071 = ( UpperDeckHeight - PanHeight ) + PanHeight - DeckThick"
equation "d2073 = ( BaseX ) + ( ( ( ( TowerWidth ) - ( 14 * SlotPitch + SlotWidth ) ) / 2 ) + ( 4 * SlotPitch ) )"
equation "d2074 = ( BaseY ) + ( Wall + DeckClearance + RimBorder )"
equation "d2075 = SlotWidth"
equation "d2076 = ( Depth ) - 2 * ( Wall + DeckClearance + RimBorder )"
equation "d2077 = DeckThick"
equation "d2079 = ( UpperDeckHeight - PanHeight ) + PanHeight - DeckThick"
equation "d2081 = ( BaseX ) + ( ( ( ( TowerWidth ) - ( 14 * SlotPitch + SlotWidth ) ) / 2 ) + ( 5 * SlotPitch ) )"
equation "d2082 = ( BaseY ) + ( Wall + DeckClearance + RimBorder )"
equation "d2083 = SlotWidth"
equation "d2084 = ( Depth ) - 2 * ( Wall + DeckClearance + RimBorder )"
equation "d2085 = DeckThick"
equation "d2087 = ( UpperDeckHeight - PanHeight ) + PanHeight - DeckThick"
equation "d2089 = ( BaseX ) + ( ( ( ( TowerWidth ) - ( 14 * SlotPitch + SlotWidth ) ) / 2 ) + ( 6 * SlotPitch ) )"
equation "d2090 = ( BaseY ) + ( Wall + DeckClearance + RimBorder )"
equation "d2091 = SlotWidth"
equation "d2092 = ( Depth ) - 2 * ( Wall + DeckClearance + RimBorder )"
equation "d2093 = DeckThick"
equation "d2095 = ( UpperDeckHeight - PanHeight ) + PanHeight - DeckThick"
equation "d2097 = ( BaseX ) + ( ( ( ( TowerWidth ) - ( 14 * SlotPitch + SlotWidth ) ) / 2 ) + ( 7 * SlotPitch ) )"
equation "d2098 = ( BaseY ) + ( Wall + DeckClearance + RimBorder )"
equation "d2099 = SlotWidth"
equation "d2100 = ( Depth ) - 2 * ( Wall + DeckClearance + RimBorder )"
equation "d2101 = DeckThick"
equation "d2103 = ( UpperDeckHeight - PanHeight ) + PanHeight - DeckThick"
equation "d2105 = ( BaseX ) + ( ( ( ( TowerWidth ) - ( 14 * SlotPitch + SlotWidth ) ) / 2 ) + ( 8 * SlotPitch ) )"
equation "d2106 = ( BaseY ) + ( Wall + DeckClearance + RimBorder )"
equation "d2107 = SlotWidth"
equation "d2108 = ( Depth ) - 2 * ( Wall + DeckClearance + RimBorder )"
equation "d2109 = DeckThick"
equation "d2111 = ( UpperDeckHeight - PanHeight ) + PanHeight - DeckThick"
equation "d2113 = ( BaseX ) + ( ( ( ( TowerWidth ) - ( 14 * SlotPitch + SlotWidth ) ) / 2 ) + ( 9 * SlotPitch ) )"
equation "d2114 = ( BaseY ) + ( Wall + DeckClearance + RimBorder )"
equation "d2115 = SlotWidth"
equation "d2116 = ( Depth ) - 2 * ( Wall + DeckClearance + RimBorder )"
equation "d2117 = DeckThick"
equation "d2119 = ( UpperDeckHeight - PanHeight ) + PanHeight - DeckThick"
equation "d2121 = ( BaseX ) + ( ( ( ( TowerWidth ) - ( 14 * SlotPitch + SlotWidth ) ) / 2 ) + ( 10 * SlotPitch ) )"
equation "d2122 = ( BaseY ) + ( Wall + DeckClearance + RimBorder )"
equation "d2123 = SlotWidth"
equation "d2124 = ( Depth ) - 2 * ( Wall + DeckClearance + RimBorder )"
equation "d2125 = DeckThick"
equation "d2127 = ( UpperDeckHeight - PanHeight ) + PanHeight - DeckThick"
equation "d2129 = ( BaseX ) + ( ( ( ( TowerWidth ) - ( 14 * SlotPitch + SlotWidth ) ) / 2 ) + ( 11 * SlotPitch ) )"
equation "d2130 = ( BaseY ) + ( Wall + DeckClearance + RimBorder )"
equation "d2131 = SlotWidth"
equation "d2132 = ( Depth ) - 2 * ( Wall + DeckClearance + RimBorder )"
equation "d2133 = DeckThick"
equation "d2135 = ( UpperDeckHeight - PanHeight ) + PanHeight - DeckThick"
equation "d2137 = ( BaseX ) + ( ( ( ( TowerWidth ) - ( 14 * SlotPitch + SlotWidth ) ) / 2 ) + ( 12 * SlotPitch ) )"
equation "d2138 = ( BaseY ) + ( Wall + DeckClearance + RimBorder )"
equation "d2139 = SlotWidth"
equation "d2140 = ( Depth ) - 2 * ( Wall + DeckClearance + RimBorder )"
equation "d2141 = DeckThick"
equation "d2143 = ( UpperDeckHeight - PanHeight ) + PanHeight - DeckThick"
equation "d2145 = ( BaseX ) + ( ( ( ( TowerWidth ) - ( 14 * SlotPitch + SlotWidth ) ) / 2 ) + ( 13 * SlotPitch ) )"
equation "d2146 = ( BaseY ) + ( Wall + DeckClearance + RimBorder )"
equation "d2147 = SlotWidth"
equation "d2148 = ( Depth ) - 2 * ( Wall + DeckClearance + RimBorder )"
equation "d2149 = DeckThick"
equation "d2151 = ( UpperDeckHeight - PanHeight ) + PanHeight - DeckThick"
equation "d2153 = ( BaseX ) + ( ( ( ( TowerWidth ) - ( 14 * SlotPitch + SlotWidth ) ) / 2 ) + ( 14 * SlotPitch ) )"
equation "d2154 = ( BaseY ) + ( Wall + DeckClearance + RimBorder )"
equation "d2155 = SlotWidth"
equation "d2156 = ( Depth ) - 2 * ( Wall + DeckClearance + RimBorder )"
equation "d2157 = DeckThick"
equation "d2159 = ( UpperDeckHeight - PanHeight ) + PanHeight - DeckThick"
equation "d2161 = ( BaseX ) + ( ( TowerWidth ) / 2 - 8 mm )"
equation "d2162 = ( BaseY ) + ( ( Depth ) - Wall - DeckClearance - 4 mm )"
equation "d2165 = DeckThick"
equation "d2169 = BaseX"
equation "d2170 = BaseY"
equation "d2171 = TowerFrame"
equation "d2172 = Depth"
equation "d2173 = UpperDeckHeight - PanHeight"
equation "d2175 = BaseX"
equation "d2177 = -( -( 8 mm ) )"
equation "d2178 = ( BaseY + 12 mm )"
equation "d2179 = ( BaseY + Depth - 12 mm )"
equation "d2180 = -( -( UpperDeckHeight - PanHeight - 8 mm ) )"
equation "d2181 = TowerFrame"
equation "d2183 = UpperDeckHeight - PanHeight"
equation "d2185 = ( BaseX ) + ( ( TowerFrame - 5 mm ) / 2 )"
equation "d2186 = ( BaseY + 8 mm ) - ( 2.5 mm )"
equation "d2189 = PegHeight"
equation "d2191 = UpperDeckHeight - PanHeight"
equation "d2193 = ( BaseX ) + ( ( TowerFrame - 5 mm ) / 2 )"
equation "d2194 = ( BaseY + Depth - 8 mm ) - ( 2.5 mm )"
equation "d2197 = PegHeight"
equation "d2201 = BaseX + TowerWidth - TowerFrame"
equation "d2202 = BaseY"
equation "d2203 = TowerFrame"
equation "d2204 = Depth"
equation "d2205 = UpperDeckHeight - PanHeight"
equation "d2207 = BaseX + TowerWidth - TowerFrame"
equation "d2209 = -( -( 8 mm ) )"
equation "d2210 = ( BaseY + 12 mm )"
equation "d2211 = ( BaseY + Depth - 12 mm )"
equation "d2212 = -( -( UpperDeckHeight - PanHeight - 8 mm ) )"
equation "d2213 = TowerFrame"
equation "d2215 = UpperDeckHeight - PanHeight"
equation "d2217 = ( BaseX + TowerWidth - TowerFrame ) + ( ( TowerFrame - 5 mm ) / 2 )"
equation "d2218 = ( BaseY + 8 mm ) - ( 2.5 mm )"
equation "d2221 = PegHeight"
equation "d2223 = UpperDeckHeight - PanHeight"
equation "d2225 = ( BaseX + TowerWidth - TowerFrame ) + ( ( TowerFrame - 5 mm ) / 2 )"
equation "d2226 = ( BaseY + Depth - 8 mm ) - ( 2.5 mm )"
equation "d2229 = PegHeight"
equation "d2231 = UpperDeckHeight - PanHeight"
equation "d2233 = ( BaseX + ( TowerFrame - 5 mm ) / 2 ) - ( FitClearance )"
equation "d2234 = ( BaseY + 8 mm ) - ( 2.5 mm + FitClearance )"
equation "d2235 = 5 mm + 2 * FitClearance"
equation "d2236 = 5 mm + 2 * FitClearance"
equation "d2237 = PegHeight + 0.3 mm"
equation "d2239 = UpperDeckHeight - PanHeight"
equation "d2241 = ( BaseX + ( TowerFrame - 5 mm ) / 2 ) - ( FitClearance )"
equation "d2242 = ( BaseY + Depth - 8 mm ) - ( 2.5 mm + FitClearance )"
equation "d2243 = 5 mm + 2 * FitClearance"
equation "d2244 = 5 mm + 2 * FitClearance"
equation "d2245 = PegHeight + 0.3 mm"
equation "d2247 = UpperDeckHeight - PanHeight"
equation "d2249 = ( BaseX + TowerWidth - TowerFrame + ( TowerFrame - 5 mm ) / 2 ) - ( FitClearance )"
equation "d2250 = ( BaseY + 8 mm ) - ( 2.5 mm + FitClearance )"
equation "d2251 = 5 mm + 2 * FitClearance"
equation "d2252 = 5 mm + 2 * FitClearance"
equation "d2253 = PegHeight + 0.3 mm"
equation "d2255 = UpperDeckHeight - PanHeight"
equation "d2257 = ( BaseX + TowerWidth - TowerFrame + ( TowerFrame - 5 mm ) / 2 ) - ( FitClearance )"
equation "d2258 = ( BaseY + Depth - 8 mm ) - ( 2.5 mm + FitClearance )"
equation "d2259 = 5 mm + 2 * FitClearance"
equation "d2260 = 5 mm + 2 * FitClearance"
equation "d2261 = PegHeight + 0.3 mm"
equation "d2265 = BaseX + LeftRun + FaucetGap + RightRun + 20 mm + 0 mm"
equation "d2266 = BaseY"
equation "d2273 = ( BaseX + LeftRun + FaucetGap + RightRun + 20 mm + 0 mm ) + ( ( 24 mm - ( PegSize + 2 * ( FitClearance - 0.05 mm ) ) ) / 2 )"
equation "d2274 = BaseY + ( 24 mm - ( PegSize + 2 * ( FitClearance - 0.05 mm ) ) ) / 2"
equation "d2275 = PegSize + 2 * ( FitClearance - 0.05 mm )"
equation "d2276 = PegSize + 2 * ( FitClearance - 0.05 mm )"
equation "d2277 = PegHeight + 0.3 mm"
equation "d2281 = BaseX + LeftRun + FaucetGap + RightRun + 20 mm + 30 mm"
equation "d2282 = BaseY"
equation "d2289 = ( BaseX + LeftRun + FaucetGap + RightRun + 20 mm + 30 mm ) + ( ( 24 mm - ( PegSize + 2 * ( FitClearance ) ) ) / 2 )"
equation "d2290 = BaseY + ( 24 mm - ( PegSize + 2 * ( FitClearance ) ) ) / 2"
equation "d2291 = PegSize + 2 * ( FitClearance )"
equation "d2292 = PegSize + 2 * ( FitClearance )"
equation "d2293 = PegHeight + 0.3 mm"
equation "d2297 = BaseX + LeftRun + FaucetGap + RightRun + 20 mm + 60 mm"
equation "d2298 = BaseY"
equation "d2305 = ( BaseX + LeftRun + FaucetGap + RightRun + 20 mm + 60 mm ) + ( ( 24 mm - ( PegSize + 2 * ( FitClearance + 0.05 mm ) ) ) / 2 )"
equation "d2306 = BaseY + ( 24 mm - ( PegSize + 2 * ( FitClearance + 0.05 mm ) ) ) / 2"
equation "d2307 = PegSize + 2 * ( FitClearance + 0.05 mm )"
equation "d2308 = PegSize + 2 * ( FitClearance + 0.05 mm )"
equation "d2309 = PegHeight + 0.3 mm"
equation "FrontFootInset = 17 mm" comment "R02 front foot center inset; outer foot edge is 9 mm behind open lip"
equation "d2312 = ( FootHeight ) - 0.2 mm"
equation "d2314 = ( BaseX + TowerFrame + TowerClearance ) + ( -1 mm )"
equation "d2315 = ( BaseY ) + ( Depth )"
equation "d2316 = ( TowerWidth - 2 * ( TowerFrame + TowerClearance ) ) + 2 mm"
equation "d2317 = DrainExtension + 2 mm"
equation "d2318 = PanHeight + 0.4 mm"
equation "d2320 = ( BaseX + TowerFrame + TowerClearance ) + ( Wall )"
equation "d2322 = -( -( ( FootHeight ) + FloorMin + DrainExtension * tan(DrainSlope) + ( ( Depth ) - ( ( Depth ) - Wall - 0.1 mm ) ) * tan(DrainSlope) ) )"
equation "d2323 = ( ( BaseY ) + ( ( Depth ) - Wall - 0.1 mm ) )"
equation "d2324 = -( -( ( FootHeight ) + FloorMin + DrainExtension * tan(DrainSlope) + ( ( Depth ) - ( ( Depth ) + 1 mm ) ) * tan(DrainSlope) ) )"
equation "d2325 = ( ( BaseY ) + ( ( Depth ) + 1 mm ) )"
equation "d2326 = -( -( ( FootHeight ) + PanHeight + 1 mm ) )"
equation "d2327 = ( TowerWidth - 2 * ( TowerFrame + TowerClearance ) ) - 2 * Wall"
equation "d2329 = ( FootHeight ) + PanHeight - DeckThick"
equation "d2331 = ( BaseX + TowerFrame + TowerClearance ) + ( ( Wall ) - DeckClearance )"
equation "d2332 = ( BaseY ) + ( 10 mm - DeckClearance )"
equation "d2333 = 2 mm + 2 * DeckClearance"
equation "d2334 = 5 mm + 2 * DeckClearance"
equation "d2335 = DeckThick"
equation "d2337 = FootHeight"
equation "d2339 = ( BaseX + TowerFrame + TowerClearance ) + ( Wall )"
equation "d2340 = ( BaseY ) + ( 10 mm )"
equation "d2343 = PanHeight"
equation "d2345 = ( FootHeight ) + PanHeight - DeckThick"
equation "d2347 = ( BaseX + TowerFrame + TowerClearance ) + ( ( ( TowerWidth - 2 * ( TowerFrame + TowerClearance ) ) - Wall - 2 mm ) - DeckClearance )"
equation "d2348 = ( BaseY ) + ( 10 mm - DeckClearance )"
equation "d2349 = 2 mm + 2 * DeckClearance"
equation "d2350 = 5 mm + 2 * DeckClearance"
equation "d2351 = DeckThick"
equation "d2353 = FootHeight"
equation "d2355 = ( BaseX + TowerFrame + TowerClearance ) + ( ( TowerWidth - 2 * ( TowerFrame + TowerClearance ) ) - Wall - 2 mm )"
equation "d2356 = ( BaseY ) + ( 10 mm )"
equation "d2359 = PanHeight"
equation "d2361 = ( FootHeight ) - 0.2 mm"
equation "d2363 = ( BaseX + TowerWidth + ModuleGap ) + ( -1 mm )"
equation "d2364 = ( BaseY ) + ( Depth )"
equation "d2365 = ( LeftRun - TowerWidth - ModuleGap ) + 2 mm"
equation "d2366 = DrainExtension + 2 mm"
equation "d2367 = PanHeight + 0.4 mm"
equation "d2369 = ( BaseX + TowerWidth + ModuleGap ) + ( Wall )"
equation "d2371 = -( -( ( FootHeight ) + FloorMin + DrainExtension * tan(DrainSlope) + ( ( Depth ) - ( ( Depth ) - Wall - 0.1 mm ) ) * tan(DrainSlope) ) )"
equation "d2372 = ( ( BaseY ) + ( ( Depth ) - Wall - 0.1 mm ) )"
equation "d2373 = -( -( ( FootHeight ) + FloorMin + DrainExtension * tan(DrainSlope) + ( ( Depth ) - ( ( Depth ) + 1 mm ) ) * tan(DrainSlope) ) )"
equation "d2374 = ( ( BaseY ) + ( ( Depth ) + 1 mm ) )"
equation "d2375 = -( -( ( FootHeight ) + PanHeight + 1 mm ) )"
equation "d2376 = ( LeftRun - TowerWidth - ModuleGap ) - 2 * Wall"
equation "d2378 = ( FootHeight ) + PanHeight - DeckThick"
equation "d2380 = ( BaseX + TowerWidth + ModuleGap ) + ( ( Wall ) - DeckClearance )"
equation "d2381 = ( BaseY ) + ( 10 mm - DeckClearance )"
equation "d2382 = 2 mm + 2 * DeckClearance"
equation "d2383 = 5 mm + 2 * DeckClearance"
equation "d2384 = DeckThick"
equation "d2386 = FootHeight"
equation "d2388 = ( BaseX + TowerWidth + ModuleGap ) + ( Wall )"
equation "d2389 = ( BaseY ) + ( 10 mm )"
equation "d2392 = PanHeight"
equation "d2394 = ( FootHeight ) + PanHeight - DeckThick"
equation "d2396 = ( BaseX + TowerWidth + ModuleGap ) + ( ( ( LeftRun - TowerWidth - ModuleGap ) - Wall - 2 mm ) - DeckClearance )"
equation "d2397 = ( BaseY ) + ( 10 mm - DeckClearance )"
equation "d2398 = 2 mm + 2 * DeckClearance"
equation "d2399 = 5 mm + 2 * DeckClearance"
equation "d2400 = DeckThick"
equation "d2402 = FootHeight"
equation "d2404 = ( BaseX + TowerWidth + ModuleGap ) + ( ( LeftRun - TowerWidth - ModuleGap ) - Wall - 2 mm )"
equation "d2405 = ( BaseY ) + ( 10 mm )"
equation "d2408 = PanHeight"
equation "d2410 = ( FootHeight ) - 0.2 mm"
equation "d2412 = ( BaseX + LeftRun + FaucetGap ) + ( -1 mm )"
equation "d2413 = ( BaseY ) + ( Depth )"
equation "d2414 = ( ( RightRun - ModuleGap ) / 2 ) + 2 mm"
equation "d2415 = DrainExtension + 2 mm"
equation "d2416 = PanHeight + 0.4 mm"
equation "d2418 = ( BaseX + LeftRun + FaucetGap ) + ( Wall )"
equation "d2420 = -( -( ( FootHeight ) + FloorMin + DrainExtension * tan(DrainSlope) + ( ( Depth ) - ( ( Depth ) - Wall - 0.1 mm ) ) * tan(DrainSlope) ) )"
equation "d2421 = ( ( BaseY ) + ( ( Depth ) - Wall - 0.1 mm ) )"
equation "d2422 = -( -( ( FootHeight ) + FloorMin + DrainExtension * tan(DrainSlope) + ( ( Depth ) - ( ( Depth ) + 1 mm ) ) * tan(DrainSlope) ) )"
equation "d2423 = ( ( BaseY ) + ( ( Depth ) + 1 mm ) )"
equation "d2424 = -( -( ( FootHeight ) + PanHeight + 1 mm ) )"
equation "d2425 = ( ( RightRun - ModuleGap ) / 2 ) - 2 * Wall"
equation "d2427 = ( FootHeight ) + PanHeight - DeckThick"
equation "d2429 = ( BaseX + LeftRun + FaucetGap ) + ( ( Wall ) - DeckClearance )"
equation "d2430 = ( BaseY ) + ( 10 mm - DeckClearance )"
equation "d2431 = 2 mm + 2 * DeckClearance"
equation "d2432 = 5 mm + 2 * DeckClearance"
equation "d2433 = DeckThick"
equation "d2435 = FootHeight"
equation "d2437 = ( BaseX + LeftRun + FaucetGap ) + ( Wall )"
equation "d2438 = ( BaseY ) + ( 10 mm )"
equation "d2441 = PanHeight"
equation "d2443 = ( FootHeight ) + PanHeight - DeckThick"
equation "d2445 = ( BaseX + LeftRun + FaucetGap ) + ( ( ( ( RightRun - ModuleGap ) / 2 ) - Wall - 2 mm ) - DeckClearance )"
equation "d2446 = ( BaseY ) + ( 10 mm - DeckClearance )"
equation "d2447 = 2 mm + 2 * DeckClearance"
equation "d2448 = 5 mm + 2 * DeckClearance"
equation "d2449 = DeckThick"
equation "d2451 = FootHeight"
equation "d2453 = ( BaseX + LeftRun + FaucetGap ) + ( ( ( RightRun - ModuleGap ) / 2 ) - Wall - 2 mm )"
equation "d2454 = ( BaseY ) + ( 10 mm )"
equation "d2457 = PanHeight"
equation "d2459 = ( FootHeight ) - 0.2 mm"
equation "d2461 = ( BaseX + LeftRun + FaucetGap + ( RightRun + ModuleGap ) / 2 ) + ( -1 mm )"
equation "d2462 = ( BaseY ) + ( Depth )"
equation "d2463 = ( ( RightRun - ModuleGap ) / 2 ) + 2 mm"
equation "d2464 = DrainExtension + 2 mm"
equation "d2465 = PanHeight + 0.4 mm"
equation "d2467 = ( BaseX + LeftRun + FaucetGap + ( RightRun + ModuleGap ) / 2 ) + ( Wall )"
equation "d2469 = -( -( ( FootHeight ) + FloorMin + DrainExtension * tan(DrainSlope) + ( ( Depth ) - ( ( Depth ) - Wall - 0.1 mm ) ) * tan(DrainSlope) ) )"
equation "d2470 = ( ( BaseY ) + ( ( Depth ) - Wall - 0.1 mm ) )"
equation "d2471 = -( -( ( FootHeight ) + FloorMin + DrainExtension * tan(DrainSlope) + ( ( Depth ) - ( ( Depth ) + 1 mm ) ) * tan(DrainSlope) ) )"
equation "d2472 = ( ( BaseY ) + ( ( Depth ) + 1 mm ) )"
equation "d2473 = -( -( ( FootHeight ) + PanHeight + 1 mm ) )"
equation "d2474 = ( ( RightRun - ModuleGap ) / 2 ) - 2 * Wall"
equation "d2476 = ( FootHeight ) + PanHeight - DeckThick"
equation "d2478 = ( BaseX + LeftRun + FaucetGap + ( RightRun + ModuleGap ) / 2 ) + ( ( Wall ) - DeckClearance )"
equation "d2479 = ( BaseY ) + ( 10 mm - DeckClearance )"
equation "d2480 = 2 mm + 2 * DeckClearance"
equation "d2481 = 5 mm + 2 * DeckClearance"
equation "d2482 = DeckThick"
equation "d2484 = FootHeight"
equation "d2486 = ( BaseX + LeftRun + FaucetGap + ( RightRun + ModuleGap ) / 2 ) + ( Wall )"
equation "d2487 = ( BaseY ) + ( 10 mm )"
equation "d2490 = PanHeight"